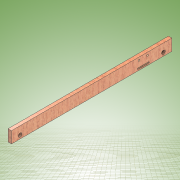
# Autodesk Inventor part: Riel_Lateral_MDF
Saved by Autodesk Inventor 2022 (Build 260153000, 153)
## iProperties
Created: 2022-02-12
Part Number: Riel_Lateral_MDF
Material: Genérico
Document SubType Name: Modeling
Designer: Marco
Density: 1 g/cm^3
Appearance: Abedul - Natural pulido
Author: Marco
Autodesk Inventor part; units mm, degrees
ref_plane "YZ Plane" through (0, 0, 0) normal (1, 0, 0) x (0, 1, 0)
ref_plane "XZ Plane" through (0, 0, 0) normal (0, 1, 0) x (-1, 0, 0)
ref_plane "XY Plane" through (0, 0, 0) normal (0, 0, 1) x (1, 0, 0)
sketch "Boceto1" plane through (0, 0, 0) normal (1, 0, 0) x (0, 1, 0)
  line L0 (0, 0) -> (20, 0)
  line L1 (20, 0) -> (20, -280)
  line L2 (20, -280) -> (0, -280)
  line L3 (0, -280) -> (0, 0)
  circle A0 centre (6, -15) radius 3.175
  circle A1 centre (6, -265) radius 3.175
  dimension "d0" = 20
  dimension "d1" = 280
  dimension "d2" = 6.35
  dimension "d8" = 6
  dimension "d9" = 250
  dimension "d10" = 15
  constraints: 8 end point, 2 centre point, 2 parallel, 1 equal radius, 1 horizontal, 1 perpendicular, 1 vertical alignment
  measures "d0" distance of L1.end L2.end
  measures "d1" distance of L2.end L0.start
  measures "d2" diameter of A0
  measures "d8" horizontal distance of L0.start A0.centre
  measures "d9" distance of A1.centre A0.centre
  measures "d10" vertical distance of L0.start A0.centre
extrude "Extrusión1" add sketch "Boceto1" along normal blind 6
sketch "Boceto2" plane through (6, 0, 0) normal (1, 0, 0) x (0, 0, -1)
  line L0 (220, 17.5) -> (240, 17.5)
  line L1 (240, 17.5) -> (240, 2.5)
  line L2 (240, 2.5) -> (220, 2.5)
  line L3 (220, 2.5) -> (220, 17.5)
  line L4 (280, 0) -> (280, 20) projected
  line L5 (240, 2.5) -> (220, 2.5)
  line L6 (220, 2.5) -> (220, 4.5)
  line L7 (220, 4.5) -> (240, 4.5)
  line L8 (240, 4.5) -> (240, 2.5)
  circle A0 centre (222.54, 14.96) radius 1.5
  line L9 (230, 17.5) -> (230, 4.5)
  circle A1 centre (237.46, 14.96) radius 1.5
  point P0 (0, 0)
  point P1 (240, 10)
  point P2 (280, 10)
  dimension "d11" = 20
  dimension "d12" = 15
  dimension "d13" = 40
  dimension "d14" = 2
  dimension "d15" = 3
  dimension "d16" = 2.54
  dimension "d17" = 2.54
  constraints: 18 end point, 4 midpoint, 4 parallel, 2 centre point, 2 horizontal, 2 perpendicular, 1 horizontal alignment, 1 point on line, 1 symmetric about line, 1 other
  measures "d11" distance of L1.end L2.end
  measures "d12" distance of L0.end L1.end
  measures "d13" distance from line of L4 L1.end
  measures "d14" distance of L2.end L6.end
  measures "d15" diameter of A0
  measures "d16" horizontal distance of L0.start A0.centre
  measures "d17" horizontal distance of L0.start A0.centre
extrude "Extrusión2" cut sketch "Boceto2" against normal through all contours L7 L1 L2 L3 | A0 | A1
